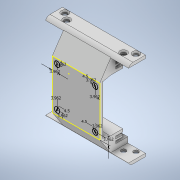
# Autodesk Inventor part: middle
Saved by Autodesk Inventor 2020 (Build 240168000, 168)
## iProperties
Created: 2021-04-17
Part Number: middle
Material: Generic
Document SubType Name: Modeling
Designer: dkiiv
Density: 1 g/cm^3
Appearance: Default
Author: dkiiv
Autodesk Inventor part; units mm, degrees
ref_plane "YZ Plane" through (0, 0, 0) normal (1, 0, 0) x (0, 1, 0)
ref_plane "XZ Plane" through (0, 0, 0) normal (0, 1, 0) x (-1, 0, 0)
ref_plane "XY Plane" through (0, 0, 0) normal (0, 0, 1) x (1, 0, 0)
sketch "Sketch1" plane through (0, 0, 0) normal (0, 0, 1) x (1, 0, 0)
  line L0 (-29.0164, 22.2951) -> (40.9836, 22.2951)
  line L1 (40.9836, 22.2951) -> (40.9836, 19.7951)
  line L2 (40.9836, 19.7951) -> (-29.0164, 19.7951)
  line L3 (-29.0164, 19.7951) -> (-29.0164, 22.2951)
  line L4 (-14.0164, 19.7951) -> (25.9836, 19.7951)
  line L5 (25.9836, 19.7951) -> (25.9836, 7.2971)
  line L6 (25.9836, 7.2971) -> (-14.0164, 7.2971)
  line L7 (-14.0164, 7.2971) -> (-14.0164, 19.7951)
  point P0 (0, 0)
  point P1 (25.9836, 19.7951)
  dimension "d0" = 70
  dimension "d1" = 2.5
  dimension "d2" = 40
  dimension "d3" = 0
  dimension "d4" = 15
  dimension "d5" = 12.498
  constraints: 16 end point, 4 parallel, 2 horizontal, 2 perpendicular
  measures "d0" distance of L0.start L0.end
  measures "d1" distance of L0.end L1.end
  measures "d2" distance of L5.end L6.end
  measures "d3" distance between parallel lines of L2 L4
  measures "d4" distance between parallel lines of L1 L5
  measures "d5" distance of L4.end L5.end
extrude "Extrusion1" add sketch "Sketch1" along normal blind 14.617
fillet "Fillet1" radius 4.074 1 edges at (5.9836, 22.2951, 14.617)
sketch "Sketch2" plane through (-29.0164, 22.2951, 0) normal (0, 1, 0) x (1, 0, 0)
  circle A0 centre (5, -3) radius 2
  circle A1 centre (11, -7.5) radius 2
  circle A2 centre (65, -3) radius 2
  circle A3 centre (59, -7.5) radius 2
  line L0 (70, 0) -> (0, 0) projected
  line L1 (0, 0) -> (0, -10.543) projected
  line L2 (70, 0) -> (70, -10.543) projected
  point P0 (29.0164, 0)
  point P1 (55, -14.617)
  point P2 (15, -14.617)
  dimension "d9" = 4
  dimension "d10" = 4
  dimension "d11" = 4
  dimension "d12" = 4
  dimension "d13" = 7.5
  dimension "d14" = 7.5
  dimension "d19" = 3
  dimension "d20" = 3
  dimension "d23" = 10
  dimension "d24" = 4
  dimension "d25" = 4
  dimension "d26" = 10
  constraints: 4 centre point
  measures "d9" diameter of A0
  measures "d10" diameter of A1
  measures "d11" diameter of A2
  measures "d12" diameter of A3
  measures "d13" distance from line of L0 A3.centre
  measures "d14" distance from line of L0 A1.centre
  measures "d19" distance from line of L0 A0.centre
  measures "d20" distance from line of L0 A2.centre
  measures "d23" horizontal distance of point (55, -14.617) A2.centre
  measures "d24" horizontal distance of point (55, -14.617) A3.centre
  measures "d25" horizontal distance of point (15, -14.617) A1.centre
  measures "d26" horizontal distance of point (15, -14.617) A0.centre
extrude "Extrusion2" cut sketch "Sketch2" against normal blind 6.633
chamfer "Chamfer1" distance 1 angle 45 4 edges at (-26.0164, 22.2951, 3) (-20.0164, 22.2951, 7.5) (27.9836, 22.2951, 7.5) (33.9836, 22.2951, 3)
sketch "Sketch3" plane through (25.9836, 7.2971, 0) normal (1, 0, 0) x (0, 0, -1)
  line L0 (0, 5.856) -> (-10.14, 5.856)
  line L1 (-10.14, 5.856) -> (-10.14, 7.856)
  line L2 (-10.14, 7.856) -> (0, 7.856)
  line L3 (0, 7.856) -> (0, 5.856)
  line L4 (0, 12.498) -> (-14.3007, 12.498) projected
  line L5 (0, 0) -> (0, 12.498) projected
  line L6 (0, 4.356) -> (-10.14, 4.356)
  line L7 (-10.14, 4.356) -> (-10.14, 2.356)
  line L8 (-10.14, 2.356) -> (0, 2.356)
  line L9 (0, 2.356) -> (0, 4.356)
  line L10 (0, 12.498) -> (0, 0) projected
  line L11 (0, 0) -> (-14.617, 0) projected
  line L12 (0, 12.498) -> (-4.14, 12.498)
  line L13 (-4.14, 12.498) -> (-4.14, 0)
  line L14 (-4.14, 0) -> (0, 0)
  line L15 (0, 0) -> (0, 12.498)
  point P0 (0, -7.2971)
  point P1 (0, 2.356)
  point P2 (0, 4.356)
  point P3 (-4.14, 2.356)
  point P4 (-4.14, 7.856)
  point P5 (-4.14, 5.856)
  point P6 (-4.14, 4.356)
  dimension "d30" = 4.642
  dimension "d31" = 0
  dimension "d32" = 10.14
  dimension "d33" = 2
  dimension "d34" = 1.5
  dimension "d35" = 0
  dimension "d36" = 10.14
  dimension "d37" = 2
  dimension "d40" = 4.14
  constraints: 24 end point, 6 parallel, 3 horizontal, 3 perpendicular, 1 point on line
  measures "d30" distance between parallel lines of L4 L2
  measures "d31" distance between parallel lines of L5 L3
  measures "d32" distance of L0.start L0.end
  measures "d33" distance of L0.end L1.end
  measures "d34" distance between parallel lines of L0 L6
  measures "d35" distance between parallel lines of L5 L9
  measures "d36" distance of L6.start L6.end
  measures "d37" distance of L6.end L7.end
  measures "d40" distance of L14.end L13.end
extrude "Extrusion4" cut sketch "Sketch3" against normal up to surface (40 mm away) contours L5 L6 L13 L0 | L0 L13 L2 L3 | L0 L1 L2 L13 | L5 L8 L13 L6 | L13 L8 L7 L6 | L5 L11 L13 L8
sketch "Sketch4" plane through (25.9836, 7.2971, 14.617) normal (1, 0, 0) x (0, 0, -1)
  arc A0 (0.3163, 12.498) -> (0, 10.924) centre (4.074, 10.924) ccw projected
  line L0 (-29.136, -25.8302) -> (13.0698, -25.8302) construction
  line L1 (-6.5, -9.8645) -> (-6.5, 25.4779) construction
  line L2 (0, 0) -> (0, 10.924) projected
  arc A1 (4.074, 14.998) -> (0.3163, 12.498) centre (4.074, 10.924) ccw projected
  line L3 (0.3163, 12.498) -> (16.8731, 12.498) construction
  line L4 (0.4718, 12.8271) -> (-6.5, 2.4519)
  line L5 (0.4718, 12.8271) -> (12.9718, 12.8271) construction
  line L6 (-9, -15.3528) -> (-9, 34.047) construction
  line L7 (-6.5, 2.4519) -> (-9, -1.2685)
  line L8 (-6.5, 2.4519) -> (-2.0177, 2.4519) construction
  line L9 (-8.403, -1.5) -> (-7.0715, -1.5) construction
  line L10 (10.477, 0) -> (0, 0) projected
  line L11 (0, 10.924) -> (0, 0) projected
  line L12 (0, 0) -> (-6.5, -1.5)
  line L13 (-9, -1.2685) -> (-9, -42.6905)
  line L14 (-9, -1.2685) -> (32.422, -1.2685) construction
  line L15 (-9, -42.6905) -> (-6.5, -42.6905) construction
  line L16 (-6.5, -42.6905) -> (-6.5, -1.5)
  line L17 (14.617, 7.856) -> (14.617, 12.498) projected
  line L18 (14.617, 7.856) -> (4.477, 7.856) projected
  line L19 (14.617, 7.856) -> (4.477, 7.856)
  line L20 (4.477, 7.856) -> (4.477, 5.856) projected
  line L21 (4.477, 7.856) -> (4.477, 5.856)
  line L22 (4.477, 5.856) -> (10.477, 5.856) projected
  line L23 (4.477, 5.856) -> (10.477, 5.856)
  line L24 (10.477, 4.356) -> (4.477, 4.356) projected
  line L25 (10.477, 5.856) -> (10.477, 4.356)
  line L26 (10.477, 4.356) -> (4.477, 4.356)
  line L27 (4.477, 4.356) -> (4.477, 2.356) projected
  line L28 (4.477, 4.356) -> (4.477, 2.356)
  line L29 (4.477, 2.356) -> (10.477, 2.356) projected
  line L30 (4.477, 2.356) -> (10.477, 2.356)
  line L31 (10.477, 2.356) -> (10.477, 0) projected
  line L32 (10.477, 2.356) -> (10.477, 0)
  line L33 (10.477, 0) -> (0, 0) projected
  line L34 (10.477, 0) -> (0, 0)
  line L35 (0, 0) -> (0, 10.924)
  line L36 (0, 10.924) -> (14.617, 10.924)
  line L37 (14.617, 7.856) -> (14.617, 10.924)
  line L38 (14.617, 12.498) -> (14.617, 14.998) projected
  line L39 (14.617, 14.998) -> (14.617, 12.498) projected
  line L40 (14.617, 10.924) -> (14.617, 14.998)
  line L41 (14.617, 14.998) -> (4.074, 14.998) projected
  line L42 (14.617, 14.998) -> (4.074, 14.998)
  arc A2 (4.074, 14.998) -> (0.3163, 12.498) centre (4.074, 10.924) ccw projected
  arc A3 (4.074, 14.998) -> (0, 10.924) centre (4.074, 10.924) ccw
  line L43 (19.3109, 14.998) -> (19.3109, -59.286) construction
  line L44 (19.3109, 14.998) -> (93.5949, 14.998) construction
  line L45 (19.3109, -22.144) -> (9.547, -22.144) construction
  arc A4 (0, -55.212) -> (0.3163, -56.786) centre (4.074, -55.212) ccw
  line L46 (0, -44.288) -> (0, -55.212)
  arc A5 (0.3163, -56.786) -> (4.074, -59.286) centre (4.074, -55.212) ccw
  line L47 (10.477, -44.288) -> (0, -44.288)
  line L48 (14.617, -52.144) -> (14.617, -56.786)
  line L49 (14.617, -52.144) -> (4.477, -52.144)
  line L50 (4.477, -52.144) -> (4.477, -50.144)
  line L51 (4.477, -50.144) -> (10.477, -50.144)
  line L52 (10.477, -48.644) -> (4.477, -48.644)
  line L53 (10.477, -50.144) -> (10.477, -48.644)
  line L54 (4.477, -48.644) -> (4.477, -46.644)
  line L55 (4.477, -46.644) -> (10.477, -46.644)
  line L56 (10.477, -46.644) -> (10.477, -44.288)
  line L57 (0, -55.212) -> (14.617, -55.212)
  line L58 (14.617, -55.212) -> (14.617, -59.286)
  line L59 (14.617, -59.286) -> (4.074, -59.286)
  line L60 (-9, -42.6905) -> (0.6662, -57.4446)
  line L61 (-6.5, -42.6905) -> (0, -44.288)
  line L62 (15.5471, -56.786) -> (-4.1669, -56.786)
  point P0 (14.617, -7.2971)
  point P1 (0.3163, -56.786)
  point P2 (0.2347, -56.786)
  point P3 (0.3163, -56.786)
  dimension "d44" = 6.5
  dimension "d46" = 123.9
  dimension "d47" = 2.5
  dimension "d48" = 123.9
  dimension "d49" = 1.5
  dimension "d50" = 41.422
  dimension "d51" = 90
  dimension "d52" = 2.5
  dimension "d53" = 90
  dimension "d59" = 74.284
  dimension "d60" = 90
  dimension "d63" = 2.5
  constraints: 96 end point, 18 symmetric about line, 10 collinear, 10 horizontal, 8 point on circle, 7 point on line, 5 perpendicular, 4 equal length, 3 centre point, 3 vertical, 1 midpoint, 1 tangent, 2 other
  measures "d44" distance between parallel lines of L2 L1
  measures "d46" angle of L4 L5
  measures "d47" distance between parallel lines of L1 L6
  measures "d48" angle of L7 L8
  measures "d49" distance between parallel lines of L10 L9
  measures "d50" distance of L7.end L13.end
  measures "d51" angle of L13 L14
  measures "d52" distance of L13.end L15.end
  measures "d53" angle of L15 L13
  measures "d59" distance of L43.start L43.end
  measures "d60" angle of L43 L44
  measures "d63" distance between parallel lines of L62 L59
extrude "Extrusion5" add sketch "Sketch4" against normal up to surface (40 mm away) contours L47 L56 L55 L54 L52 L53 L51 L50 L49 L48 L57 L46 | L57 L48 L62 A4 | A5 L62 L58 L59
extrude "Extrusion6" add sketch "Sketch4" along normal up to surface (15 mm away) contours A5 L62 L58 L59
extrude "Extrusion7" add sketch "Sketch4" against normal up to surface (55 mm away) contours A5 L62 L58 L59
extrude "Extrusion8" cut sketch "Sketch2" against normal blind 83.25
chamfer "Chamfer2" distance 1 angle 45 4 edges at (-20.0164, -51.9889, 7.5) (-26.0164, -51.9889, 3) (27.9836, -51.9889, 7.5) (33.9836, -51.9889, 3)
extrude "Extrusion9" add sketch "Sketch4" against normal up to surface (40 mm away) contours A0 L2 L12 L16 L61 L46 A4 L62 L60 L13 L7 L4 A1
sketch "Sketch5" plane through (25.9836, -35.3934, 23.617) normal (0, 0, 1) x (1, 0, 0)
  circle A0 centre (-36.038, 37.46) radius 2.25
  circle A1 centre (-3.962, 37.46) radius 2.25
  circle A2 centre (-36.038, 3.962) radius 2.25
  circle A3 centre (-3.962, 3.962) radius 2.25
  line L0 (0, 41.422) -> (-40, 41.422) projected
  line L1 (-40, 41.422) -> (-40, 0) projected
  line L2 (0, 41.422) -> (0, 0) projected
  line L3 (0, 0) -> (-40, 0) projected
  point P0 (-25.9836, 35.3934)
  dimension "d75" = 4.5
  dimension "d76" = 4.5
  dimension "d77" = 4.5
  dimension "d78" = 4.5
  dimension "d79" = 3.962
  dimension "d80" = 3.962
  dimension "d81" = 3.962
  dimension "d82" = 3.962
  dimension "d83" = 3.962
  dimension "d84" = 3.962
  dimension "d85" = 3.962
  dimension "d86" = 3.962
  constraints: 4 centre point
  measures "d75" diameter of A0
  measures "d76" diameter of A1
  measures "d77" diameter of A2
  measures "d78" diameter of A3
  measures "d79" distance from line of L0 A0.centre
  measures "d80" distance from line of L1 A0.centre
  measures "d81" distance from line of L0 A1.centre
  measures "d82" distance from line of L2 A1.centre
  measures "d83" distance from line of L2 A3.centre
  measures "d84" distance from line of L3 A3.centre
  measures "d85" distance from line of L3 A2.centre
  measures "d86" distance from line of L1 A2.centre
body "Solid1"
